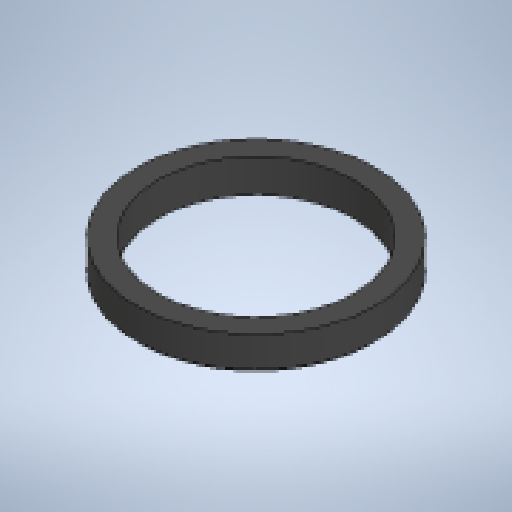
# Autodesk Inventor part: Band
Saved by Autodesk Inventor 2023.2 (Build 272271000, 271)
## iProperties
Created: 2023-06-16
Part Number: Band
Material: Rubber, Silicone
Document SubType Name: Modeling
Designer: Nathan Cai
Density: 1.25 g/cm^3
Appearance: Rubber - Black
Author: Nathan Cai
Autodesk Inventor part; units mm, degrees
ref_plane "YZ Plane" through (0, 0, 0) normal (1, 0, 0) x (0, 1, 0)
ref_plane "XZ Plane" through (0, 0, 0) normal (0, 1, 0) x (-1, 0, 0)
ref_plane "XY Plane" through (0, 0, 0) normal (0, 0, 1) x (1, 0, 0)
sketch "Sketch1" plane through (0, 0, 0) normal (0, 1, 0) x (-1, 0, 0)
  circle A0 centre (0, 0) radius 21.8281 construction
  circle A1 centre (0, 0) radius 18.6531
  circle A2 centre (0, 0) radius 22.225 construction
  circle A3 centre (0, 0) radius 22.725
  dimension "d0" = 43.6562
  dimension "d1" = 3.175
  dimension "d2" = 44.45
  dimension "d3" = 0.5
  constraints: 4 centre point, 3 coincident
  measures "d0" diameter of A0
  measures "d1" radial gap between concentric circles of A0 A1
  measures "d2" diameter of A2
  measures "d3" radial gap between concentric circles of A2 A3
extrude "Extrusion1" add sketch "Sketch1" along normal blind 6.35
chamfer "Chamfer1" distance 0.5 angle 45 1 edges at (22.725, 0, 0)
body "Solid1"
